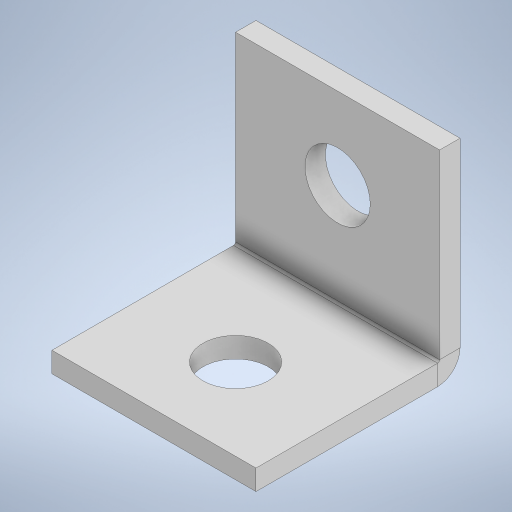
# Autodesk Inventor part: connector
Saved by Autodesk Inventor 2023 (Build 270158000, 158)
## iProperties
Created: 2023-05-25
Part Number: connector
Material: 一般
Document SubType Name: Sheet Metal
Designer: 310611102
Density: 1 g/cm^3
Sheet Metal Rule: Default_mm
Appearance: 預設
Author: 310611102
Autodesk Inventor part; units mm, degrees
ref_plane "YZ Plane" through (0, 0, 0) normal (1, 0, 0) x (0, 1, 0)
ref_plane "XZ Plane" through (0, 0, 0) normal (0, 1, 0) x (-1, 0, 0)
ref_plane "XY Plane" through (0, 0, 0) normal (0, 0, 1) x (1, 0, 0)
sketch "Sketch1" plane through (0, 0, 0) normal (0, 0, 1) x (1, 0, 0)
  line L0 (-5, 5) -> (5, 5)
  line L1 (5, 5) -> (5, -5)
  line L2 (5, -5) -> (-5, -5)
  line L3 (-5, -5) -> (-5, 5)
  line L4 (-5, 5) -> (5, -5) construction
  line L5 (5, 5) -> (-5, -5) construction
  circle A0 centre (0, 1) radius 1.6
  point P0 (0, 0)
  dimension "d0" = 10
  dimension "d1" = 10
  dimension "d3" = 3.2
  dimension "d21" = 4
  measures "d0" distance of L0.end L1.end
  measures "d1" distance of L0.start L0.end
  measures "d3" diameter of A0
  measures "d21" distance from line of L0 A0.centre
extrude "Plate1" add sketch "Sketch1" along normal blind 1
sketch "Sketch2" plane through (5, -4, 0) normal (0, -1, 0) x (1, 0, 0)
  line L0 (-10, 0) -> (0, 0)
  line L1 (0, 0) -> (0, 10)
  line L2 (0, 10) -> (-10, 10)
  line L3 (-10, 10) -> (-10, 0)
  constraints: 6 end point, 1 horizontal, 1 perpendicular, 1 vertical
edge flange "Flange1" height 10 angle 90 thickness 1 bend radius 0.1 thickness toward (0, -1, 0) relief straight relief width 1 relief depth 0.5 edges at (0, -5, 1) wall of the first edge with corners at (-5, -4, 0) (5, -4, 0) (5, -4, 10) (-5, -4, 10)
bend "Bend1"
corner "Corner1"
sketch "Sketch3" plane through (-5, -4, 10) normal (0, 1, 0) x (1, 0, 0)
  circle A0 centre (5, 4) radius 1.6
  line L0 (0, 9) -> (10, 9) projected
  line L1 (0, 0) -> (10, 0) projected
  point P0 (5, 10)
  point P1 (5, 0)
  dimension "d17" = 3.2
  dimension "d22" = 4
  constraints: 1 centre point, 1 midpoint, 1 vertical alignment
  measures "d17" diameter of A0
  measures "d22" distance from line of A0.centre L1
extrude "Cut1" cut sketch "Sketch3" against normal blind 1
equation "\"d19\" = 厚度"
equation "\"d6\" = 厚度"
equation "\"d7\" = 折彎離隙寬度"
equation "\"d8\" = 折彎離隙深度"
equation "\"d9\" = 最小剩餘"
equation "\"d10\" = 轉移半徑"
equation "\"d14\" = 轉角離隙大小"
equation "\"d15\" = 間隙大小"
equation "\"d16\" = Jacobi半徑大小"
equation "\"折彎半徑\" = 厚度"
equation "\"折彎離隙寬度\" = 厚度"
equation "\"折彎離隙深度\" = 0.5 * 厚度"
equation "\"轉角離隙大小\" = 4 * 厚度"
equation "\"最小剩餘\" = 2 * 厚度"
equation "\"轉移半徑\" = 折彎半徑"
equation "\"Jacobi半徑大小\" = 折彎半徑"
equation "\"間隙大小\" = 厚度"
equation "\"厚度\" = 1"
body "Solid1"
